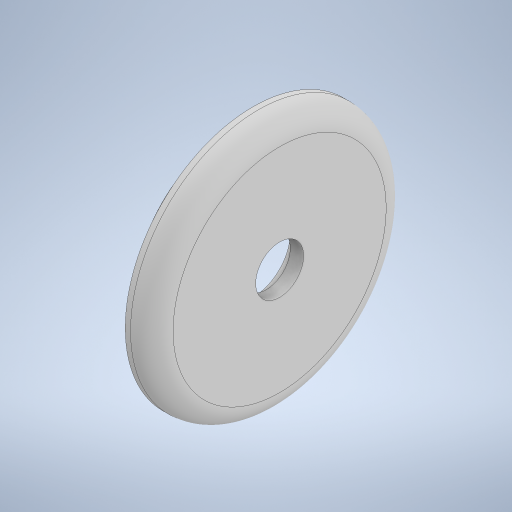
# Autodesk Inventor part: Parte2
Saved by Autodesk Inventor 2024 (Build 280153000, 153)
## iProperties
Created: 2024-02-26
Part Number: Parte2
Material: Generico
Document SubType Name: Modeling
Designer: Leonardo
Density: 1 g/cm^3
Appearance: Default
Author: Leonardo
Autodesk Inventor part; units mm, degrees
ref_plane "YZ Plane" through (0, 0, 0) normal (1, 0, 0) x (0, 1, 0)
ref_plane "XZ Plane" through (0, 0, 0) normal (0, 1, 0) x (-1, 0, 0)
ref_plane "XY Plane" through (0, 0, 0) normal (0, 0, 1) x (1, 0, 0)
sketch "Schizzo3" plane through (0, 0, 0) normal (0, 1, 0) x (-1, 0, 0)
  line L0 (0, 0) -> (-2.5, 0)
  line L1 (-2.5, 0) -> (-2.5, -12)
  line L2 (-2.5, -12) -> (0, -12)
  line L3 (0, -12) -> (0, -9.2831)
  line L4 (0, -9.2831) -> (1.9415, -9.2831)
  line L5 (1.9415, -9.2831) -> (1.9415, -7.7495)
  line L6 (1.9415, -7.7495) -> (0, -7.7495)
  line L7 (0, -7.7495) -> (0, 0)
  line L8 (1.9415, -9.2831) -> (1.133, -9.9738)
  line L9 (1.133, -9.9738) -> (1.133, -9.2831)
  dimension "d5" = 2.5
  dimension "d6" = 12
  constraints: 20 end point, 8 perpendicular, 2 point on line, 1 horizontal
  measures "d5" distance of L0.start L0.end
  measures "d6" distance of L0.end L1.end
revolve "Rivoluzione1" add sketch "Schizzo3" angle 360 about axis through (0, 0, 0) along (1, 0, 0)
fillet "Raccordo1" radius 2 1 edges at (2.5, 0, 12)
sketch "Schizzo6" plane through (0, 0, 0) normal (-1, 0, 0) x (0, 0, 1)
  point P0 (0, 0)
  point P1 (0, 0)
  constraints: 1 coincident
hole "Foro1" at (0, 0, 0) direction (1, 0, 0) diameter 4.5 depth 8 countersink diameter 7 countersink angle 90
